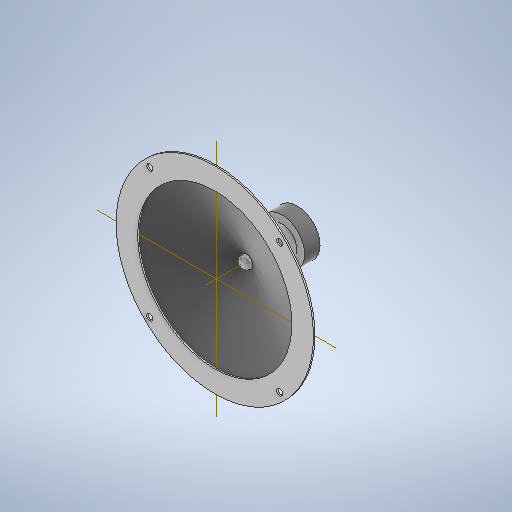
# Autodesk Inventor part: 스피커
Saved by Autodesk Inventor 2025.1 (Build 291241000, 241)
## iProperties
Created: 2024-10-28
Part Number: 스피커
Material: 일반
Document SubType Name: Modeling
Designer: gmsee
Density: 1 g/cm^3
Appearance: 기본값
Author: gmsee
Autodesk Inventor part; units mm, degrees
ref_plane "YZ Plane" through (0, 0, 0) normal (1, 0, 0) x (0, 1, 0)
ref_plane "XZ Plane" through (0, 0, 0) normal (0, 1, 0) x (-1, 0, 0)
ref_plane "XY Plane" through (0, 0, 0) normal (0, 0, 1) x (1, 0, 0)
sketch "스케치1" plane through (0, 0, 0) normal (0, 0, 1) x (1, 0, 0)
  circle A0 centre (0, 0) radius 64
  circle A1 centre (42.072, 42.072) radius 2
  line L0 (-89.6, 0) -> (89.6, 0) projected
  line L1 (0, -89.6) -> (0, 89.6) projected
  circle A2 centre (-42.072, 42.072) radius 2
  circle A3 centre (-42.072, -42.072) radius 2
  circle A4 centre (42.072, -42.072) radius 2
  circle A5 centre (0, 0) radius 50
  dimension "d0" = 128
  dimension "d1" = 4
  dimension "d2" = 42.072
  dimension "d3" = 42.072
  dimension "d4" = 4
  dimension "d5" = 4
  dimension "d6" = 4
  dimension "d7" = 42.072
  dimension "d8" = 42.072
  dimension "d9" = 42.072
  dimension "d10" = 42.072
  dimension "d11" = 42.072
  dimension "d12" = 42.072
  dimension "d15" = 100
  constraints: 6 centre point, 2 coincident
  measures "d0" diameter of A0
  measures "d1" diameter of A1
  measures "d2" distance from line of L0 A1.centre
  measures "d3" distance from line of A1.centre L1
  measures "d4" diameter of A2
  measures "d5" diameter of A3
  measures "d6" diameter of A4
  measures "d7" distance from line of L1 A2.centre
  measures "d8" distance from line of L0 A2.centre
  measures "d9" distance from line of L0 A3.centre
  measures "d10" distance from line of L1 A3.centre
  measures "d11" distance from line of A4.centre L0
  measures "d12" distance from line of L1 A4.centre
  measures "d15" diameter of A5
extrude "돌출1" add sketch "스케치1" along normal blind 1 contours L0 A5 L1 A0 | A0 L1 A5 L0 | L1 A5 L0 A0 | A0 L0 A5 L1
sketch "스케치4" plane through (0, 0, 0) normal (0, 1, 0) x (-1, 0, 0)
  line L0 (0, -15.9722) -> (0, -52.5)
  line L1 (0, -52.5) -> (-14.78, -52.5)
  line L2 (-14.78, -52.5) -> (-14.78, -42.5)
  line L3 (64, 0) -> (-64, 0) projected
  line L4 (-14.78, -42.5) -> (-9.78, -42.5)
  line L5 (-50, 0) -> (50, 0) projected
  line L6 (-9.78, -42.5) -> (-50, 0)
  line L7 (-50, 0) -> (0, 0)
  line L8 (-50, 0) -> (-4.1334, -19.5682)
  arc A0 (0, -15.9722) -> (-4.1334, -19.5682) centre (0.1079, -20.2698) ccw
  line L9 (0, -63.2) -> (0, 11.7) projected
  dimension "d16" = 52.5
  dimension "d17" = 14.78
  dimension "d18" = 10
  dimension "d19" = 5
  dimension "d20" = 20
  constraints: 14 end point, 2 horizontal, 2 point on circle, 2 vertical, 1 centre point, 1 collinear, 1 midpoint
  measures "d16" distance of L7.end L0.end
  measures "d17" distance of L0.end L1.end
  measures "d18" distance of L1.end L2.end
  measures "d19" distance of L2.end L4.end
  measures "d20" distance of point (0, 0) L8.end
revolve "회전1" add sketch "스케치4" angle 360 about axis through (0, 0, -10) along (0, 0, 1) contours L0 L1 L2 L4 L6 L8 A0
